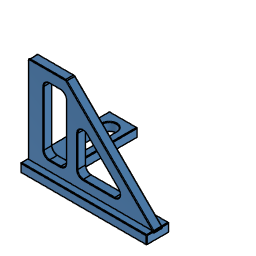
Week 2_Task 2_Square_Ohene (Autodesk Fusion 360 design; units mm, degrees)
Autodesk Fusion 360 part; units mm, degrees
note: some values were not read from the file. Set by a fixed rule: which sketch regions a step uses.
sketch "Vertical Piece" plane through (0, 0, 0) normal (0, 1, 0) x (1, 0, 0)
  line L0 (1.5, 0) -> (110.75, 0)
  line L1 (111.5, -0.75) -> (111.5, -1.1888)
  line L2 (33.1798, -79) -> (1.5, -79)
  line L3 (0, -77.5) -> (0, -1.5)
  line L4 (0, -60) -> (13.8, -60) construction
  line L5 (13.8, -79) -> (13.8, 0) construction
  line L6 (13.8, -66.3956) -> (33.8, -66.3956) construction
  line L7 (33.8, -64) -> (33.8, 0) construction
  line L8 (0, -1.5) -> (111.5, -1.5) construction
  line L9 (28.8, -69) -> (0, -69) construction
  line L10 (18.8, -69) -> (33.8, -69)
  line L11 (33.8, -69) -> (33.8, -15)
  line L12 (28.8, -10) -> (18.8, -10)
  line L13 (13.8, -15) -> (13.8, -64)
  arc A0 (18.8, -10) -> (13.8, -15) centre (18.8, -15) ccw
  arc A1 (33.8, -15) -> (28.8, -10) centre (28.8, -15) ccw
  arc A2 (13.8, -64) -> (18.8, -69) centre (18.8, -64) ccw
  arc A3 (28.8, -69) -> (33.8, -64) centre (28.8, -64) ccw
  arc A4 (0, -77.5) -> (1.5, -79) centre (1.5, -77.5) ccw
  arc A5 (1.5, 0) -> (0, -1.5) centre (1.5, -1.5) ccw
  line L14 (43.8, -42.8527) -> (43.8, -15)
  line L15 (28.8, -10) -> (30.7692, -10)
  line L16 (48.8, -10) -> (76.7246, -10)
  line L17 (34.2391, -78.562) -> (111.2796, -1.7198)
  arc A6 (111.5, -0.75) -> (110.75, 0) centre (110.75, -0.75) ccw
  arc A7 (111.2796, -1.7198) -> (111.5, -1.1888) centre (110.75, -1.1888) ccw
  line L18 (52.331, -46.3928) -> (80.2555, -18.5401)
  arc A8 (43.8, -42.8527) -> (52.331, -46.3928) centre (48.8, -42.8527) ccw
  arc A9 (80.2555, -18.5401) -> (76.7246, -10) centre (76.7246, -15) ccw
  arc A10 (48.8, -10) -> (43.8, -15) centre (48.8, -15) ccw
  arc A11 (33.1798, -79) -> (34.2391, -78.562) centre (33.1798, -77.5) ccw
  line L19 (0, -79) -> (111.5, -79)
  line L20 (111.5, -79) -> (111.5, 0)
  line L21 (111.5, 0) -> (0, 0)
  line L22 (0, 0) -> (0, -79)
  point P0 (111.5, 0)
  point P1 (0, -79)
  point P2 (13.8, -69)
  point P3 (13.8, -10)
  dimension "d8" = 111.5
  dimension "d9" = 79
  dimension "d11" = 13.8
  dimension "d12" = 20
  dimension "d16" = 59
  dimension "d18" = 5
  dimension "d19" = 5
  dimension "d20" = 5
  dimension "d21" = 5
  dimension "d24" = 1.5
  dimension "d25" = 1.5
  dimension "d27" = 0.75
  dimension "d28" = 0.75
  dimension "d30" = 5
  dimension "d31" = 5
  dimension "d32" = 5
  dimension "d33" = 1.5
  constraint horizontal L0
  constraint vertical L1
  constraint horizontal L2
  constraint vertical L3
  constraint coincident L21.end L22.start
  constraint coincident L3 L4.start
  constraint perpendicular L3 L4
  constraint coincident L0 L5.end
  constraint perpendicular L0 L5
  constraint coincident L2 L5.start
  constraint coincident L4.end L5
  constraint coincident L5 L6.start
  constraint perpendicular L5 L6
  constraint coincident L0 L7.end
  constraint perpendicular L0 L7
  constraint coincident L6.end L7
  constraint horizontal L10
  constraint vertical L11
  constraint horizontal L12
  constraint vertical L13
  constraint coincident L5 P2
  constraint coincident L9 P2
  constraint coincident P3 L12
  constraint coincident P3 L13
  constraint tangent L12 A0
  constraint tangent L13 A0
  constraint tangent L12 A1
  constraint tangent L11 A1
  constraint coincident P2 L13
  constraint coincident P2 L10
  constraint tangent L13 A2
  constraint tangent L10 A2
  constraint tangent L9 A3
  constraint tangent L7 A3
  constraint coincident P0 L0
  constraint coincident P0 L1
  constraint coincident P1 L3
  constraint coincident P1 L2
  constraint tangent L3 A4
  constraint tangent L2 A4
  constraint coincident L21.end L3
  constraint coincident L21.end L0
  constraint tangent L3 A5
  constraint tangent L0 A5
  constraint tangent A1 L15
  constraint perpendicular L7 L16
  constraint tangent L0 A6
  constraint tangent L1 A6
  constraint coincident L8.end L17
  constraint tangent L17 A7
  constraint tangent L1 A7
  constraint tangent L14 A8
  constraint tangent L18 A8
  constraint tangent L16 A9
  constraint tangent L18 A9
  constraint coincident L15.end L16
  constraint tangent L14 A10
  constraint tangent L16 A10
  constraint tangent L2 A11
  constraint tangent L17 A11
  constraint horizontal L19
  constraint vertical L20
  constraint horizontal L21
  constraint vertical L22
  constraint coincident P0 L20.end
  constraint coincident P1 L19.start
  measures "d8" distance of L21.end P0
  measures "d9" distance of L21.end L19.start
  measures "d11" distance of L4.start L4.end
  measures "d12" distance of L6.start L6.end
  measures "d16" distance of P2 P3
  measures "d18" radius of A0
  measures "d19" radius of A1
  measures "d20" radius of A2
  measures "d21" radius of A3
  measures "d24" radius of A4
  measures "d25" radius of A5
  measures "d27" radius of A6
  measures "d28" radius of A7
  measures "d30" radius of A8
  measures "d31" radius of A9
  measures "d32" radius of A10
  measures "d33" radius of A11
extrude "Extrude1" add sketch "Vertical Piece" along normal blind 3.9 and the other way blind 3.9 contours L0 L1 L2 L3 A4 A5 L17 A6 A7 A11 L19 L20 L21 L22 | L10 L11 A3 makes body 1
extrude "Extrude2" add sketch "Vertical Piece" along normal blind 3.9 and the other way blind 3.9 separate body contours L0 L1 L2 L3 A4 A5 L17 A6 A7 A11 L19 L20 L21 L22 | A5 L21 L22 | A6 L20 L21 | A4 L19 L22 | L17 A7 A11 L19 L20 | L10 L11 L12 L13 A0 A1 A2 A3 | L10 L11 A3 | L14 L16 L18 A8 A9 A10 makes body 2
sketch "Horizontal Piece" plane through (0, 0, 0) normal (0, 0, -1) x (1, 0, 0)
  line L0 (0, 3.9) -> (0, -3.9)
  line L1 (0, -3.9) -> (111.5, -3.9)
  line L2 (111.5, -3.9) -> (111.5, 3.9)
  line L3 (111.5, 3.9) -> (0, 3.9)
  line L4 (111.5, -3.9) -> (0, 3.9) construction
  line L5 (55.75, 0) -> (130, 0) construction
  line L6 (111.5, 0) -> (111.5, 10)
  line L7 (111.5, 10) -> (-0.5, 10)
  line L8 (-0.5, 10) -> (-0.5, -69)
  line L9 (-0.5, -69) -> (24.5, -69)
  line L10 (24.5, -69) -> (24.5, 40)
  line L11 (111.5, -10) -> (-0.5, -10)
  line L12 (111.5, 0) -> (111.5, -10)
  line L13 (5.8, 10) -> (5.8, -69)
  line L14 (18.2, -69) -> (18.2, 40)
  line L15 (-0.5, -62.7) -> (24.5, -62.7) construction
  line L16 (5.8, -50.3) -> (18.2, -50.3) construction
  line L17 (18.2, -50.3) -> (5.8, -62.7) construction
  circle A0 centre (12, -56.5) radius 6.2
  line L18 (12, -62.7) -> (12, -22.7) construction
  line L19 (12, -42.7) -> (18.2, -42.7) construction
  circle A1 centre (12, -28.9) radius 6.2
  line L20 (0, -3.9) -> (-0.5, -3.9)
  line L21 (0, 3.9) -> (-0.5, 3.9)
  circle A2 centre (24.5, -10) radius 4.1
  dimension "d48" = 10
  dimension "d49" = 112
  dimension "d50" = 79
  dimension "d51" = 25
  dimension "d52" = -6.3
  dimension "d53" = -6.3
  dimension "d54" = -6.3
  dimension "d55" = 40
  dimension "d61" = 8.2
  constraint coincident L1.end L2.start
  constraint coincident L0.start L3.end
  constraint midpoint L4 L5.start
  constraint parallel L1 L5
  constraint midpoint L2 L6.start
  constraint perpendicular L5 L6
  constraint perpendicular L6 L7
  constraint perpendicular L7 L8
  constraint perpendicular L8 L9
  constraint perpendicular L7 L10
  constraint symmetric L5 L6.end L11.start
  constraint symmetric L5 L7.end L11.end
  constraint coincident L13 L16.start
  constraint coincident L14 L16.end
  constraint midpoint L17 A0.centre
  constraint tangent L15 A0
  constraint midpoint L15 L18.start
  constraint perpendicular L15 L18
  constraint midpoint L18 L19.start
  constraint coincident L14 L19.end
  constraint perpendicular L14 L19
  constraint symmetric A0 L19 A1
  constraint coincident L0.end L1.start
  constraint coincident L8 L20.end
  constraint perpendicular L8 L20
  constraint coincident L8 L21.end
  constraint perpendicular L8 L21
  constraint coincident L11 A2.centre
  constraint coincident L10 A2.centre
  measures "d48" distance of L6.start L6.end
  measures "d49" distance of L6.end L7.end
  measures "d50" distance of L7.end L8.end
  measures "d51" distance of L8.end L9.end
  measures "d55" distance of L18.start L18.end
  measures "d61" diameter of A2
extrude "Extrude3" add sketch "Horizontal Piece" against normal blind 1.5 separate body contours L3 L7 L8 L13 L21 | L1 L8 L11 L13 L20 | L3 L7 L13 L14 | L1 L11 L13 L14 | L3 L7 L10 L14 | L1 L10 L11 L14 A2 | L8 L9 L11 L13 | L11 L13 L14 A1 | L3 L6 L7 L10 | L1 L10 L11 L12 A2 | L9 L10 L11 L14 A2 | L10 L11 A2 | L10 L11 A2 | L10 L11 A2 | L9 L13 L14 A0 picked at (24.6945, -7.2806) picked at (21.7806, -9.8055) picked at (23.5472, -12.5545) makes body 3 at (11.8456, 12.2058, 0) makes body 4 at (36.8333, -7.9667, 0)
extrude "Extrude4" add sketch "Horizontal Piece" along normal blind 6.3 separate body contours L0 L1 L3 L13 | L3 L7 L8 L13 L21 | L0 L8 L20 L21 | L1 L8 L11 L13 L20 | L3 L7 L13 L14 | L1 L3 L13 L14 | L1 L11 L13 L14 | L3 L7 L10 L14 | L1 L3 L10 L14 | L1 L10 L11 L14 A2 | L8 L9 L11 L13 | L11 L13 L14 A1 | L3 L6 L7 L10 | L1 L2 L3 L6 L10 L12 | L1 L10 L11 L12 A2 | L9 L10 L11 L14 A2 | L10 L11 A2 | L10 L11 A2 | L10 L11 A2 | L9 L13 L14 A0 picked at (24.6945, -7.2806) picked at (21.7806, -9.8055) picked at (23.5472, -12.5545) makes body 5
combine "Combine1" operation add target body 3 tool bodies 4 5
extrude "Extrude5" cut sketch "Horizontal Piece" along normal blind 19 contours L10 L11 A2 | L10 L11 A2 | L10 L11 A2 | L10 L11 A2 bodies 3
extrude "Extrude6" cut sketch "Horizontal Piece" against normal blind 6 contours L10 L11 A2 | L10 L11 A2 | L10 L11 A2 | L10 L11 A2 bodies 3
fillet "Fillet1" radius 0.5 2 faces at (4.6, 3.9, 31.3333) (4.6, -3.9, 31.3333) on bodies 1
fillet "Fillet2" radius 0.5 9 faces at (18.2, 47.3, -3.7) (9.45, 23.2487, -3.7) (5.8, 47.3, -1.1) (6.2868, 58.9083, -1.1) (7.8333, 69, -3.7) (24.5, 32.4, -1.1) (28.5951, 9.7988, -3.7) (83.8667, 10, -3.7) (36.8333, -10, -3.7) on bodies 3
fillet "Fillet3" radius 0.5 2 edges at (111.3536, -9.8536, 1.3536) (111.5, -6.7, 1.5) on bodies 3
fillet "Fillet4" radius 0.5 2 edges at (111.5, 6.7, 1.5) (111.3536, 9.8536, 1.3536) on bodies 3
fillet "Fillet5" radius 0.5 3 edges at (111.3536, 9.8536, -6.1536) (111.5, 0, -6.3) (111.3536, -9.8536, -6.1536) on bodies 3
fillet "Fillet6" radius 0.5 7 edges at (-0.3536, 68.8536, 1.3536) (-0.5, 36.2, 1.5) (-0.5, -6.7, 1.5) (-0.3536, -9.8536, 1.3536) (-0.3536, -9.8536, -6.1536) (-0.5, 29.5, -6.3) (-0.3536, 68.8536, -6.1536) on bodies 3
hidden bodies 2
equation "Vertical_Length = 111.5 mm"
equation "Vertical_Height = 79 mm"
equation "Vertical_Depth = 7.8 mm"
equation "Vertical_Hole_1_T_Offset = 10 mm"
equation "Vertical_Hole_1_Width = 20 mm"
equation "Vertical_Hole_1_Height = 59 mm"
equation "Vertical_Hole_1_S_Offset = 13.8 mm"
equation "d8 = Vertical_Length"
equation "d9 = Vertical_Height"
equation "d11 = Vertical_Hole_1_S_Offset"
equation "d12 = Vertical_Hole_1_Width"
equation "Vertical_Hole_1_Fillet_1 = 1.5 mm"
equation "d16 = Vertical_Hole_1_Height"
equation "Vertical_Hole_1_Fillet_2 = 5 mm"
equation "d19 = Vertical_Hole_1_Fillet_2"
equation "d21 = Vertical_Hole_1_Fillet_2"
equation "d24 = Vertical_Hole_1_Fillet_1"
equation "d25 = Vertical_Hole_1_Fillet_1"
equation "d27 = Vertical_Hole_1_Fillet_1 / 2"
equation "d28 = Vertical_Hole_1_Fillet_1 / 2"
equation "d30 = Vertical_Hole_1_Fillet_2"
equation "d31 = Vertical_Hole_1_Fillet_2"
equation "d32 = Vertical_Hole_1_Fillet_2"
equation "d33 = Vertical_Hole_1_Fillet_1"
equation "d34 = Vertical_Depth / 2"
equation "d36 = Vertical_Depth / 2"
equation "Edge_Fillet = 0.5 mm"
equation "d39 = Vertical_Depth / 2"
equation "d41 = Vertical_Depth / 2"
equation "Horizontal_F_1_Width = 20 mm"
equation "Horizontal_F_2_Width = 25 mm"
equation "Horizontal_F_2_Length = 79 mm"
equation "Horizontal_F_2_Hole_S_Offset = 6.3 mm"
equation "Horizontal_F_2_Hole_Length = 40 mm"
equation "d48 = Vertical_Hole_1_Width / 2"
equation "d49 = Vertical_Length + 0.5 mm"
equation "d50 = Horizontal_F_2_Length"
equation "d51 = Horizontal_F_2_Width"
equation "d52 = -Horizontal_F_2_Hole_S_Offset"
equation "d53 = -Horizontal_F_2_Hole_S_Offset"
equation "d54 = -Horizontal_F_2_Hole_S_Offset"
equation "d55 = Horizontal_F_2_Hole_Length"
equation "d56 = -Vertical_Hole_1_Fillet_1"
equation "d58 = Vertical_Depth - Vertical_Hole_1_Fillet_1"
equation "Horizontal_H_2_Diameter = 8.2 mm"
equation "d67 = Edge_Fillet"
equation "d69 = Edge_Fillet"
equation "d71 = Edge_Fillet"
equation "d73 = Edge_Fillet"
equation "d75 = Edge_Fillet"
equation "d77 = Edge_Fillet"
